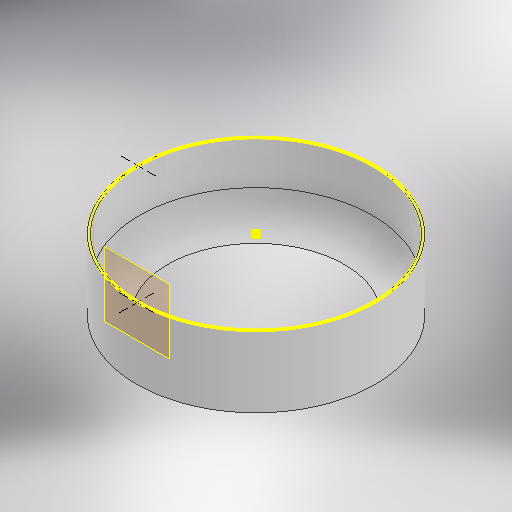
# Autodesk Inventor part: ridge_v2_treads
Saved by Autodesk Inventor 2026 (Build 300175050, 175E)
## iProperties
Created: 2026-06-28
Part Number: ridge_v2_treads
Material: Generic
Document SubType Name: Modeling
Designer: satom
Density: 1 g/cm^3
Appearance: Default
Author: satom
Autodesk Inventor part; units mm, degrees
ref_plane "YZ Plane" through (0, 0, 0) normal (1, 0, 0) x (0, 1, 0)
ref_plane "XZ Plane" through (0, 0, 0) normal (0, 1, 0) x (-1, 0, 0)
ref_plane "XY Plane" through (0, 0, 0) normal (0, 0, 1) x (1, 0, 0)
sketch "Sketch1" plane through (0, 0, 0) normal (0, 1, 0) x (-1, 0, 0)
  circle A0 centre (0, 0) radius 39.75
  circle A1 centre (0, 0) radius 40.5
  dimension "d0" = 79.5
  dimension "d1" = 81
  constraints: 2 centre point, 2 coincident
  measures "d0" diameter of A0
  measures "d1" diameter of A1
extrude "Extrusion1" add sketch "Sketch1" along normal blind 24
sketch "Sketch3" plane through (0, 24, 0) normal (0, 1, 0) x (1, 0, 0)
  circle A0 centre (0, 0) radius 40.5 projected
  circle A1 centre (0, 0) radius 39.75 projected
  point P0 (0, -40.5)
  point P1 (-39.75, 0)
  constraints: 1 horizontal alignment, 1 vertical alignment, 2 other
ref_plane "Work Plane2" through (0, 24, 40.5) normal (0, 0, 1) x (1, 0, 0)
sketch "Sketch8" plane through (0, 24, 40.5) normal (0, 0, 1) x (1, 0, 0)
  line L0 (40.5, -24) -> (40.5, 0) construction
  line L1 (40.5, -12) -> (-39.75, -12) construction
  line L2 (-39.75, 0) -> (-39.75, -24) construction
  line L3 (40.5, 0) -> (-40.5, 0) projected
  line L4 (10, 0) -> (0, 0)
  line L5 (10, -8) -> (10, 0)
  line L6 (40.5, -24) -> (-40.5, -24) projected
  line L7 (10, -16) -> (10, -24)
  line L8 (10, -24) -> (0, -24)
  line L9 (0, 0) -> (0, -8)
  line L10 (0, -8) -> (10, -8)
  line L11 (0, -24) -> (0, -16)
  line L12 (0, -16) -> (10, -16)
  point P0 (0, -24)
  point P1 (-5, -12)
  point P2 (1, -12)
  point P3 (0, 0)
  dimension "d46" = 8
  dimension "d47" = 8
  dimension "d48" = 10
  dimension "d49" = 10
  dimension "d50" = 8
  dimension "d51" = 0
  dimension "d52" = 0
  constraints: 18 end point, 4 midpoint, 4 point on line, 2 perpendicular, 2 vertical, 1 horizontal, 1 parallel
  measures "d46" distance of L5.start L4.start
  measures "d47" distance of L4.end L9.end
  measures "d48" distance of L9.end L5.start
  measures "d49" distance of L11.end L7.start
  measures "d50" distance of L7.start L7.end
  measures "d51" distance from line of point (0, -24) L11
  measures "d52" distance from line of point (0, 0) L9
emboss "Emboss3" [suppressed]
sketch "Sketch7" plane through (0, 0, 0) normal (0, 0, 1) x (1, 0, 0)
  line L0 (39.75, 24) -> (39.75, 0) construction
  line L1 (0, 0) -> (-30, 0) construction
  line L2 (0, 0) -> (0, 12) construction
  line L3 (0, 12) -> (-39.75, 12) construction
  line L4 (0, 24) -> (-30, 24) construction
  ellipse E0 centre (0, 0.5748) end of major axis (-20.7169, 56.9851) minor radius 37.0729 (-40.5, 24) -> (-40.231, 12) ccw projected
  line L5 (-30, 0) -> (-40.5, 0)
  line L6 (-40.5, 24) -> (-40.5, 0)
  line L7 (-40.5, 12) -> (-37.9524, 12) construction
  line L8 (-40.5, 12) -> (-40.5, 13.6344) construction
  arc A0 (-39.6019, 9.6019) -> (-30, 0) centre (-30, 9.6019) ccw
  line L9 (-30, 0) -> (-30, 9.6019) construction
  line L10 (-39.6019, 9.6019) -> (-30, 9.6019) construction
  line L11 (-30, 24) -> (-30, 13.1677) construction
  line L12 (-40.8323, 13.1677) -> (-30, 13.1677) construction
  line L13 (0, -7.1864) -> (0, 29.1977) projected
  line L14 (-39.6019, 9.6019) -> (-39.6019, 0)
  point P0 (-39.5989, 9.3602)
  dimension "d24" = 30
  dimension "d25" = 12
  dimension "d26" = 39.75
  dimension "d27" = 30
  dimension "d28" = 90
  dimension "d29" = 90
  constraints: 26 end point, 3 horizontal, 3 point on line, 2 perpendicular, 2 point on circle, 2 vertical, 1 centre point, 1 midpoint, 1 tangent, 1 other
  measures "d24" distance of L1.start L1.end
  measures "d25" distance of L1.start L2.end
  measures "d26" distance of L2.end L3.end
  measures "d27" distance of L4.start L4.end
  measures "d28" angle of L10 L9
  measures "d29" angle of L11 L12
revolve "Revolution1" add sketch "Sketch7" angle 360 about axis through (0, -10, 0) along (0, 1, 0)
pattern_circular "Circular Pattern4" [suppressed]
equation "\"d47\" = d46"
body "Solid1"
